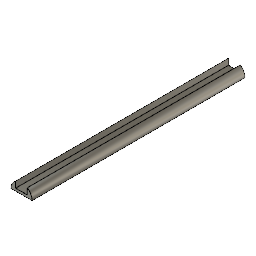
Front_pannel_holder v1 (Autodesk Fusion 360 design; units mm, degrees)
Autodesk Fusion 360 part; units mm, degrees
sketch "Sketch1" plane through (0, 0, 0) normal (0, 1, 0) x (1, 0, 0)
  arc A0 (-2, 0) -> (2, 0) centre (0, 0) ccw
  line L0 (-2, 0) -> (2, 0)
  dimension "d1" = 4
  measures "d1" distance of A0.start A0.end
extrude "Extrude1" add sketch "Sketch1" along normal blind 40
sketch "Sketch2" plane through (0, 0, 0) normal (0, -1, 0) x (1, 0, 0)
  arc A0 (2, 0) -> (-2, 0) centre (0, 0) ccw
  line L0 (-2, 0) -> (2, 0)
  line L1 (-1.1, 0.5) -> (1.1, 0.5)
  line L2 (1.1, 0.5) -> (1.1, 3.5)
  line L3 (1.1, 3.5) -> (-1.1, 3.5)
  line L4 (-1.1, 3.5) -> (-1.1, 0.5)
  line L5 (-1.1, 0.5) -> (1.1, 3.5) construction
  line L6 (1.1, 0.5) -> (-1.1, 3.5) construction
  point P0 (0, 2)
  dimension "d4" = 2.2
  dimension "d5" = 3
  measures "d4" distance of L2.end L3.end
  measures "d5" distance of L1.end L2.end
extrude "Extrude2" cut sketch "Sketch2" against normal blind 40 contours A0 L1 L2 L4
